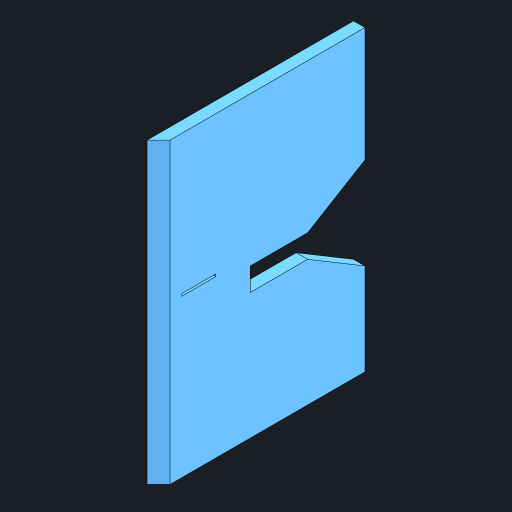
# Autodesk Inventor part: VertMove
Saved by Autodesk Inventor 2023 (Build 270158000, 158)
## iProperties
Created: 2022-06-07
Part Number: VertMove
Material: スタイロフォームIB
Document SubType Name: Modeling
Designer: neko2
Density: 0.027 g/cm^3
Appearance: スタイロフォームIB
Author: neko2
Autodesk Inventor part; units mm, degrees
ref_plane "YZ Plane" through (0, 0, 0) normal (1, 0, 0) x (0, 1, 0)
ref_plane "XZ Plane" through (0, 0, 0) normal (0, 1, 0) x (-1, 0, 0)
ref_plane "XY Plane" through (0, 0, 0) normal (0, 0, 1) x (1, 0, 0)
sketch "スケッチ1" plane through (0, 0, 0) normal (1, 0, 0) x (0, 1, 0)
  line L0 (-65, 20) -> (65, 20)
  line L1 (65, 20) -> (65, -20)
  line L2 (65, -20) -> (-65, -20)
  line L3 (-65, -20) -> (-65, 20)
  line L4 (-65, 20) -> (65, -20) construction
  line L5 (65, 20) -> (-65, -20) construction
  line L6 (65, -20) -> (65, -70)
  line L7 (65, -70) -> (15, -70)
  line L8 (15, -70) -> (0, -45)
  line L9 (-10, -45) -> (-25, -70)
  line L10 (-25, -70) -> (-65, -70)
  line L11 (-65, -70) -> (-65, -20)
  line L12 (0, -45) -> (-10, -45)
  line L13 (0, -20) -> (-10, -20)
  line L14 (-10, -20) -> (-10, -45)
  line L15 (-10, -45) -> (0, -45)
  line L16 (0, -45) -> (0, -20)
  point P0 (0, 0)
  point P1 (-5, -45)
  point P2 (0, 0)
  point P3 (0, -45)
  dimension "d0" = 130
  dimension "d1" = 40
  dimension "d18" = 50
  dimension "d19" = 50
  dimension "d22" = 5
  dimension "d24" = 25
  dimension "d25" = 10
  constraints: 34 end point, 5 midpoint, 5 parallel, 4 perpendicular, 3 horizontal, 1 collinear, 1 equal length, 1 vertical
  measures "d0" distance of L1.end L2.end
  measures "d1" distance of L0.end L1.end
  measures "d18" distance of L1.end L6.end
  measures "d19" distance of L6.end L7.end
  measures "d22" horizontal distance of point (-5, -45) point (0, 0)
  measures "d24" distance of L9.start L13.end
  measures "d25" distance of L9.start L8.end
extrude "押し出し1" add sketch "スケッチ1" along normal blind 5 contours L0 L1 L2 L3 | L2 L14 L9 L10 L11 | L6 L7 L8 L16 L2
sketch "スケッチ3" plane through (5, 0, 0) normal (1, 0, 0) x (0, 0, -1)
  line L0 (-10, 3.5) -> (5, 3.5)
  line L1 (5, 3.5) -> (5, 4.5)
  line L2 (5, 4.5) -> (-10, 4.5)
  line L3 (-10, 4.5) -> (-10, 3.5)
  line L4 (-15, 0) -> (10, 0)
  line L5 (10, 0) -> (10, 8)
  line L6 (10, 8) -> (-15, 8)
  line L7 (-15, 8) -> (-15, 0)
  line L8 (-20, 65) -> (-20, -65) projected
  point P0 (0, 0)
  point P1 (-2.5, 8)
  point P2 (-2.5, 4.5)
  point P3 (-10, 4)
  point P4 (-15, 4)
  dimension "d7" = 15
  dimension "d8" = 1
  dimension "d9" = 25
  dimension "d10" = 8
  dimension "d17" = 5
  constraints: 16 end point, 4 midpoint, 4 parallel, 2 horizontal, 2 perpendicular, 1 horizontal alignment, 1 point on line, 1 vertical alignment
  measures "d7" distance of L2.end L1.end
  measures "d8" distance of L1.end L0.end
  measures "d9" distance of L5.end L6.end
  measures "d10" distance of L4.end L5.end
  measures "d17" distance between parallel lines of L8 L7
extrude "押し出し3" cut sketch "スケッチ3" against normal through all contours L3 L2 L1 L0
chamfer "面取り1" distance 5 angle 45 1 edges at (5, 0, 20)
